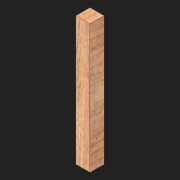
# Autodesk Inventor part: C009
Saved by Autodesk Inventor 2017 SP1 (Build 210196100, 196)
## iProperties
Created: 2017-06-14
Part Number: C009
Material: Wood (Birch)
Document SubType Name: Modeling
Designer: zallen
Density: 0.55 g/cm^3
Appearance: Birch - Natural Polished
Description: 174.5 mm
Author: zallen
Autodesk Inventor part; units mm, degrees
ref_plane "YZ Plane" through (0, 0, 0) normal (1, 0, 0) x (0, 1, 0)
ref_plane "XZ Plane" through (0, 0, 0) normal (0, 1, 0) x (-1, 0, 0)
ref_plane "XY Plane" through (0, 0, 0) normal (0, 0, 1) x (1, 0, 0)
sketch "Sketch2" plane through (0, 0, 0) normal (0, 0, 1) x (1, 0, 0)
  line L0 (0, 0) -> (19.05, 0)
  line L1 (19.05, 0) -> (19.05, 174.5)
  line L2 (19.05, 174.5) -> (0, 174.5)
  line L3 (0, 174.5) -> (0, 0)
  dimension "d9" = 19.05
  dimension "d10" = 174.5
  constraints: 8 end point, 2 parallel, 1 horizontal, 1 perpendicular
  measures "d9" distance of L2.end L1.end
  measures "d10" distance of L1.end L0.end
extrude "Extrusion1" add sketch "Sketch2" along normal blind 19.05
body "Solid1"
